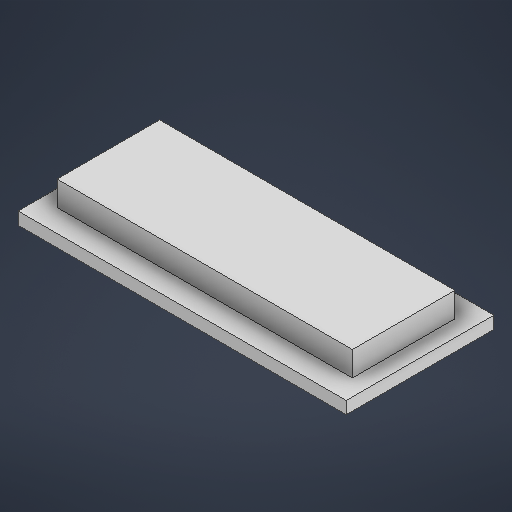
# Autodesk Inventor part: display
Saved by Autodesk Inventor 2025.2 (Build 292293000, 293)
## iProperties
Created: 2024-12-17
Part Number: display
Material: Generic
Document SubType Name: Modeling
Designer: antem
Density: 1 g/cm^3
Appearance: Default
Author: antem
Autodesk Inventor part; units mm, degrees
ref_plane "YZ Plane" through (0, 0, 0) normal (1, 0, 0) x (0, 1, 0)
ref_plane "XZ Plane" through (0, 0, 0) normal (0, 1, 0) x (-1, 0, 0)
ref_plane "XY Plane" through (0, 0, 0) normal (0, 0, 1) x (1, 0, 0)
sketch "Sketch1" plane through (0, 0, 0) normal (0, 0, 1) x (1, 0, 0)
  line L0 (-40, 18) -> (40, 18)
  line L1 (40, 18) -> (40, -18)
  line L2 (40, -18) -> (-40, -18)
  line L3 (-40, -18) -> (-40, 18)
  line L4 (-36, 12.5) -> (36, 12.5)
  line L5 (36, 12.5) -> (36, -12.5)
  line L6 (36, -12.5) -> (-36, -12.5)
  line L7 (-36, -12.5) -> (-36, 12.5)
  point P0 (0, 0)
  point P1 (-40, 0)
  point P2 (-36, 0)
  point P3 (0, 18)
  point P4 (0, 12.5)
  dimension "d0" = 36
  dimension "d1" = 80
  dimension "d2" = 25
  dimension "d3" = 72
  constraints: 16 end point, 4 midpoint, 4 parallel, 2 horizontal, 2 horizontal alignment, 2 perpendicular, 2 vertical alignment
  measures "d0" distance of L0.end L1.end
  measures "d1" distance of L0.start L0.end
  measures "d2" distance of L4.end L5.end
  measures "d3" distance of L4.start L4.end
extrude "Extrusion1" add sketch "Sketch1" against normal blind 3 contours L0 L1 L2 L3 | L4 L5 L6 L7
extrude "Extrusion2" add sketch "Sketch1" along normal blind 6 contours L4 L5 L6 L7
body "Solid1"
